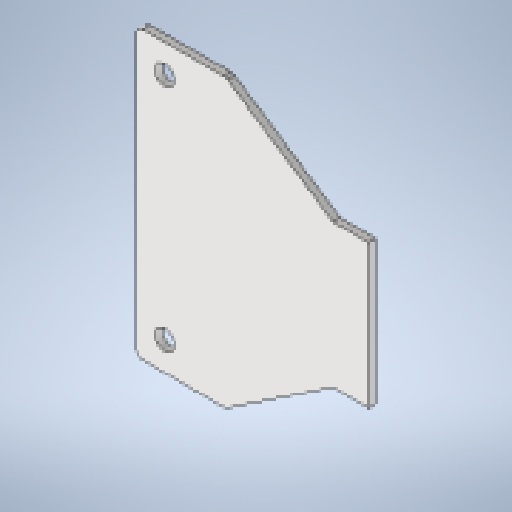
# Autodesk Inventor part: NDM 7.46 bracket floor stringer
Saved by Autodesk Inventor 2025 (Build 290162010, 162A)
## iProperties
Part Number: NDM 7.46 bracket floor stringer
Sheet Metal Rule: Default_mm
Autodesk Inventor part; units mm, degrees
ref_plane "YZ Plane" through (0, 0, 0) normal (1, 0, 0) x (0, 1, 0)
ref_plane "XZ Plane" through (0, 0, 0) normal (0, 1, 0) x (-1, 0, 0)
ref_plane "XY Plane" through (0, 0, 0) normal (0, 0, 1) x (1, 0, 0)
sketch "Sketch13" plane through (0, 0, 0) normal (0, 0, 1) x (1, 0, 0)
  line L0 (-25, -40) -> (-25, 40)
  line L1 (-25, 40) -> (0, 40)
  line L2 (0, 40) -> (30, 20)
  line L3 (30, -20) -> (0, -40)
  line L4 (0, -40) -> (-25, -40)
  line L5 (30, 20) -> (40, 20)
  line L6 (40, 20) -> (40, -20)
  line L7 (40, -20) -> (30, -20)
  line L8 (30, -20) -> (30, 20) construction
  circle A0 centre (-17, 32) radius 2.75
  circle A1 centre (-17, -32) radius 2.75
  line L9 (-25, 0) -> (30, 0) construction
  point P0 (0, 0)
  point P1 (40, 0)
  dimension "d95" = 25
  dimension "d96" = 80
  dimension "d97" = 40
  dimension "d98" = 10
  dimension "d100" = 5.5
  dimension "d101" = 8
  dimension "d102" = 8
  dimension "d103" = 30
  measures "d95" distance from line of L0 point (0, 0)
  measures "d96" distance of L0.start L0.end
  measures "d97" distance of L2.end L3.start
  measures "d98" distance of L5.start L5.end
  measures "d100" diameter of A0
  measures "d101" distance from line of A0.centre L0
  measures "d102" distance from line of A0.centre L1
  measures "d103" distance from line of point (0, 0) L8
extrude "Plate5" add sketch "Sketch13" along normal blind 2
fillet "Fillet4" radius 2 4 edges at (-25, 40, 1) (0, 40, 1) (0, -40, 1) (-25, -40, 1)
equation "\"d104\" = Thickness"
equation "\"BendRadius\" = Thickness"
equation "\"BendReliefWidth\" = Thickness"
equation "\"BendReliefDepth\" = 0.5 * Thickness"
equation "\"CornerReliefSize\" = 4 * Thickness"
equation "\"MinimumRemnant\" = 2 * Thickness"
equation "\"TransitionRadius\" = BendRadius"
equation "\"JacobiRadiusSize\" = BendRadius"
equation "\"GapSize\" = Thickness"
equation "\"Thickness\" = 2"
body "Solid2"
